test (Autodesk Fusion 360 design; units mm, degrees)
Autodesk Fusion 360 part; units mm, degrees
sketch "Sketch1" plane through (0, 0, 0) normal (0, 0, 1) x (1, 0, 0)
  line L0 (-185.5036, 143.2023) -> (197.9033, 143.2023)
  line L1 (197.9033, 143.2023) -> (197.9033, 31.9807)
  line L2 (197.9033, 31.9807) -> (-185.5036, 31.9807)
  line L3 (-185.5036, 31.9807) -> (-185.5036, 143.2023)
  line L4 (-509.3458, -1.7289) -> (543.0785, -1.7289)
  line L5 (543.0785, -1.7289) -> (543.0785, 12.2929)
  line L6 (543.0785, 12.2929) -> (-509.3458, 12.2929)
  line L7 (-509.3458, 12.2929) -> (-509.3458, -1.7289)
  line L8 (-176.6396, -37.6024) -> (201.0979, -37.6024)
  line L9 (201.0979, -37.6024) -> (201.0979, -191.7031)
  line L10 (201.0979, -191.7031) -> (-176.6396, -191.7031)
  line L11 (-176.6396, -191.7031) -> (-176.6396, -37.6024)
  constraint horizontal L0
  constraint vertical L1
  constraint horizontal L2
  constraint vertical L3
  constraint horizontal L4
  constraint vertical L5
  constraint horizontal L6
  constraint vertical L7
  constraint horizontal L8
  constraint vertical L9
  constraint horizontal L10
  constraint vertical L11
extrude "Extrude1" add sketch "Sketch1" along normal blind 10 contours L0 L1 L2 L3 | L8 L9 L10 L11 makes body 1 at (-57.7013, 106.1284, 0) makes body 2 at (-50.7271, -140.3362, 0)
extrude "Extrude2" add sketch "Sketch1" along normal mid plane 490.148 separate body contours L4 L5 L6 L7 makes body 3
